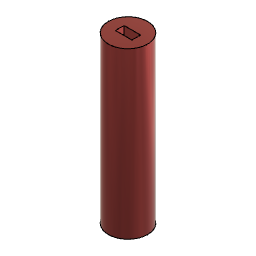
toolbox-handle (Autodesk Fusion 360 design; units mm, degrees)
Autodesk Fusion 360 part; units mm, degrees
sketch "Sketch1" plane through (0, 0, 0) normal (0, 1, 0) x (1, 0, 0)
  circle A0 centre (0, 0) radius 12.5
  dimension "d1" = 25
  constraint coincident A0.centre origin
  measures "d1" diameter of A0
extrude "Extrude1" add sketch "Sketch1" along normal blind 105
sketch "Sketch2" plane through (0, 105, 0) normal (0, 1, 0) x (-1, 0, 0)
  circle A0 centre (0, 0) radius 12.5
  line L0 (-5.25, -2.75) -> (5.25, -2.75)
  line L1 (5.25, -2.75) -> (5.25, 2.75)
  line L2 (5.25, 2.75) -> (-5.25, 2.75)
  line L3 (-5.25, 2.75) -> (-5.25, -2.75)
  line L4 (-5.25, -2.75) -> (5.25, 2.75) construction
  line L5 (5.25, -2.75) -> (-5.25, 2.75) construction
  dimension "d4" = 10.5
  dimension "d5" = 5.5
  constraint horizontal L0
  constraint perpendicular L0 L1
  constraint parallel L0 L2
  constraint parallel L1 L3
  constraint coincident L4 A0.centre
  constraint coincident L5 A0.centre
  constraint coincident A0.centre origin
  measures "d4" distance of L1.end L2.end
  measures "d5" distance of L0.end L1.end
extrude "Extrude2" cut sketch "Sketch2" against normal blind 8 contours L0 L1 L2 L3
sketch "Sketch3" plane through (0, 0, 0) normal (0, -1, 0) x (1, 0, 0)
  circle A0 centre (0, 0) radius 12.5
extrude "Extrude3" cut sketch "Sketch2" along normal blind 8 from surface at -105 contours L0 L1 L2 L3
